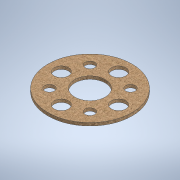
# Autodesk Inventor part: Anillo de Soporte
Saved by Autodesk Inventor 2020 (Build 240168000, 168)
## iProperties
Created: 2021-09-30
Part Number: Anillo de Soporte
Material: MDF Medium Density Fiberboard
Document SubType Name: Modeling
Designer: Carlos
Density: 0.8 g/cm^3
Appearance: Cardboard - Corrugated
Mass: 5.44354 g
Surface Area: 68.2458 cm^2
Volume: 6.80443 cm^3
Author: Carlos
Autodesk Inventor part; units mm, degrees
ref_plane "YZ Plane" through (0, 0, 0) normal (1, 0, 0) x (0, 1, 0)
ref_plane "XZ Plane" through (0, 0, 0) normal (0, 1, 0) x (-1, 0, 0)
ref_plane "XY Plane" through (0, 0, 0) normal (0, 0, 1) x (1, 0, 0)
sketch "Sketch1" plane through (0, 0, 0) normal (0, 1, 0) x (-1, 0, 0)
  circle A0 centre (0, 0) radius 35.17
  circle A1 centre (0, 0) radius 12.75
  dimension "d0" = 70.34
  dimension "d1" = 25.5
  constraints: 2 centre point, 2 coincident
  measures "d0" diameter of A0
  measures "d1" diameter of A1
extrude "Extrusion1" add sketch "Sketch1" along normal blind 2.5
sketch "Sketch2" plane through (0, 2.5, 0) normal (0, 1, 0) x (1, 0, 0)
  circle A0 centre (0, 0) radius 12.75 projected
  line L0 (12.75, 0) -> (34.4208, 0)
  line L1 (0, 12.75) -> (0, 35.17)
  circle A1 centre (0, 0) radius 35.17 projected
  circle A2 centre (0, 23.96) radius 6
  circle A3 centre (-23.96, 0) radius 6
  circle A4 centre (0, -23.96) radius 6
  circle A5 centre (23.96, 0) radius 6
  line L2 (0, 0) -> (31, 31)
  line L3 (0, 0) -> (43.8406, 0) construction
  circle A6 centre (0, 0) radius 23.96
  circle A7 centre (16.9423, 16.9423) radius 4
  circle A8 centre (-16.9423, 16.9423) radius 4
  circle A9 centre (-16.9423, -16.9423) radius 4
  circle A10 centre (16.9423, -16.9423) radius 4
  dimension "d4" = 12
  dimension "d7" = 360
  dimension "d9" = 45
  dimension "d10" = 8
  dimension "d13" = 360
  constraints: 9 centre point, 8 end point, 4 point on circle, 2 coincident, 2 horizontal, 1 equal length, 1 midpoint, 1 point on line, 1 vertical, 1 vertical alignment, 19 other
  measures "d4" diameter of A2
  measures "d9" angle of L3 L2
  measures "d10" diameter of A7
extrude "Extrusion2" cut sketch "Sketch2" against normal blind 10 contours A2 A6 L1 | L1 A6 A2 | A5 A6 L0 | L0 A6 A5 | A7 A6 L2 | L2 A6 A7 | A6 A2 L1 | L1 A2 A6 | A6 A5 L0 | L0 A5 A6 | A6 A7 L2 | L2 A7 A6 | A8 A6 | A6 A8 | A10 A6 | A6 A10 | A6 A3 | A3 A6 | A6 A4 | A4 A6 | A9 A6 | A6 A9
body "Solid1"
